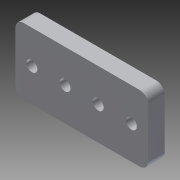
# Autodesk Inventor part: Spacer 3
Saved by Autodesk Inventor 2014 SP1 (Build 180222100, 222)
## iProperties
Created: 2014-01-14
Part Number: Spacer 3
Material: Aluminum 6061
Document SubType Name: Modeling
Designer: Arpan
Density: 2.71 g/cm^3
Appearance: Aluminum - Flat
Author: Arpan
Autodesk Inventor part; units mm, degrees
ref_plane "YZ Plane" through (0, 0, 0) normal (1, 0, 0) x (0, 1, 0)
ref_plane "XZ Plane" through (0, 0, 0) normal (0, 1, 0) x (-1, 0, 0)
ref_plane "XY Plane" through (0, 0, 0) normal (0, 0, 1) x (1, 0, 0)
sketch "Sketch1" plane through (0, 0, 0) normal (0, 0, 1) x (1, 0, 0)
  line L0 (3.175, 0) -> (47.625, 0)
  line L1 (50.8, 3.175) -> (50.8, 22.225)
  line L2 (47.625, 25.4) -> (3.175, 25.4)
  line L3 (0, 22.225) -> (0, 3.175)
  circle A0 centre (6.35, 12.7) radius 2.0701
  circle A1 centre (31.75, 12.7) radius 2.0701
  arc A2 (3.175, 25.4) -> (0, 22.225) centre (3.175, 22.225) ccw
  arc A3 (50.8, 22.225) -> (47.625, 25.4) centre (47.625, 22.225) ccw
  arc A4 (47.625, 0) -> (50.8, 3.175) centre (47.625, 3.175) ccw
  arc A5 (0, 3.175) -> (3.175, 0) centre (3.175, 3.175) ccw
  circle A6 centre (19.05, 12.7) radius 2.0701
  circle A7 centre (44.45, 12.7) radius 2.0701
  point P0 (0, 0)
  point P1 (50.8, 25.4)
  point P2 (50.8, 0)
  point P3 (0, 25.4)
  dimension "d0" = 50.8
  dimension "d1" = 25.4
  dimension "d2" = 4.1402
  dimension "d3" = 12.7
  dimension "d4" = 6.35
  dimension "d7" = 25.4
  dimension "d21" = 3.175
  dimension "d25" = 4.1402
  dimension "d26" = 12.7
  dimension "d27" = 12.7
  dimension "d30" = 25.4
  constraints: 8 centre point, 8 end point, 8 point on circle, 8 point on line, 8 tangent, 3 equal radius, 3 horizontal, 2 parallel, 1 perpendicular, 4 other
  measures "d0" distance of point (0, 25.4) point (50.8, 25.4)
  measures "d1" distance of point (50.8, 25.4) point (50.8, 0)
  measures "d2" diameter of A0
  measures "d3" distance from line of L0 A0.centre
  measures "d4" distance from line of L3 A0.centre
  measures "d7" distance of A0.centre A1.centre
  measures "d21" radius of A2
  measures "d25" diameter of A6
  measures "d26" distance from line of L0 A6.centre
  measures "d27" distance of A0.centre A6.centre
  measures "d30" distance of A6.centre A7.centre
extrude "Extrusion1" add sketch "Sketch1" along normal blind 6.35
body "Solid1"
